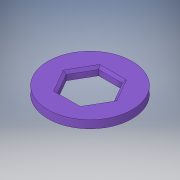
# Autodesk Inventor part: spacerForEndV03
Saved by Autodesk Inventor 2019.3 (Build 233278000, 278)
## iProperties
Created: 2019-03-05
Part Number: spacerForEndV03
Material: PC/ABS Plastic
Document SubType Name: Modeling
Designer: steele
Density: 0.357273 g/cm^3
Appearance: Violet
Author: steele
Autodesk Inventor part; units mm, degrees
ref_plane "YZ Plane" through (0, 0, 0) normal (1, 0, 0) x (0, 1, 0)
ref_plane "XZ Plane" through (0, 0, 0) normal (0, 1, 0) x (-1, 0, 0)
ref_plane "XY Plane" through (0, 0, 0) normal (0, 0, 1) x (1, 0, 0)
sketch "Sketch1" plane through (0, 0, 0) normal (0, 1, 0) x (-1, 0, 0)
  circle A0 centre (0, 0) radius 31.75
  dimension "od" = 63.5
  constraints: 1 centre point, 1 coincident
  measures "od" diameter of A0
extrude "Extrusion1" add sketch "Sketch1" against normal blind 2.54
sketch "Sketch2" plane through (0, 0, 0) normal (0, 1, 0) x (1, 0, 0)
  line L0 (-7.7063, 0) -> (-3.8531, 6.6738)
  line L1 (-3.8531, 6.6738) -> (3.8531, 6.6738)
  line L2 (3.8531, 6.6738) -> (7.7063, 0)
  line L3 (7.7063, 0) -> (3.8531, -6.6738)
  line L4 (3.8531, -6.6738) -> (-3.8531, -6.6738)
  line L5 (-3.8531, -6.6738) -> (-7.7063, 0)
  point P0 (0, 0)
  point P1 (0, 0)
  dimension "d3" = 13.3477
  constraints: 12 end point, 1 coincident, 1 horizontal, 13 other
  measures "d3" distance between parallel lines of L4 L1
extrude "Extrusion2" cut sketch "Sketch2" against normal through all
chamfer "Chamfer1" distance 0.7937 angle 45 6 edges at (-5.7797, 0, -3.3369) (0, 0, -6.6738) (5.7797, 0, -3.3369) (5.7797, 0, 3.3369) (0, 0, 6.6738) (-5.7797, 0, 3.3369)
sketch "Sketch4" plane through (0, -2.54, 0) normal (0, -1, 0) x (1, 0, 0)
  circle A0 centre (0, 0) radius 13.589
  circle A1 centre (0, 0) radius 31.75
  constraints: 2 centre point, 2 coincident
extrude "Extrusion4" cut sketch "Sketch4" against normal through all
body "Solid1"
